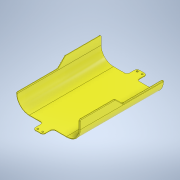
# Autodesk Inventor part: Cover_Inferior
Saved by Autodesk Inventor 2020 (Build 240168000, 168)
## iProperties
Created: 2021-06-25
Part Number: Cover_Inferior
Material: Plástico PC/ABS
Document SubType Name: Modeling
Designer: JCarlos
Density: 0.357273 g/cm^3
Appearance: Amarelo
Author: JCarlos
Autodesk Inventor part; units mm, degrees
ref_plane "YZ Plane" through (0, 0, 0) normal (1, 0, 0) x (0, 1, 0)
ref_plane "XZ Plane" through (0, 0, 0) normal (0, 1, 0) x (-1, 0, 0)
ref_plane "XY Plane" through (0, 0, 0) normal (0, 0, 1) x (1, 0, 0)
sketch "Esboço1" plane through (0, 0, 0) normal (0, 0, 1) x (1, 0, 0)
  line L0 (-62.5, 0) -> (-62.5, -10)
  line L1 (-37.5, -35) -> (37.5, -35)
  line L2 (62.5, -10) -> (62.5, 0)
  arc A0 (37.5, -35) -> (62.5, -10) centre (37.5, -10) ccw
  arc A1 (-62.5, -10) -> (-37.5, -35) centre (-37.5, -10) ccw
  line L3 (37.5, -37) -> (-37.5, -37)
  arc A2 (-64.5, -10) -> (-37.5, -37) centre (-37.5, -10) ccw
  line L4 (-64.5, -10) -> (-64.5, 0)
  line L5 (64.5, 0) -> (64.5, -10)
  arc A3 (37.5, -37) -> (64.5, -10) centre (37.5, -10) ccw
  line L6 (-64.5, 0) -> (-62.5, 0)
  line L7 (62.5, 0) -> (64.5, 0)
  point P0 (0, 0)
  point P1 (0, 0)
  point P2 (0, -35)
  dimension "d0" = 125
  dimension "d2" = 25
  dimension "d21" = 2
  dimension "d22" = 37
  dimension "d23" = 2
  dimension "d24" = 2
  dimension "d25" = 2
  dimension "d26" = 2
  constraints: 16 end point, 8 point on circle, 4 centre point, 4 tangent, 2 horizontal, 2 perpendicular, 1 coincident, 1 collinear, 1 equal radius, 1 horizontal alignment, 1 midpoint, 1 vertical alignment, 1 other
  measures "d0" distance between parallel lines of L0 L2
  measures "d2" radius of A0
  measures "d21" distance between parallel lines of L1 L3
  measures "d22" distance between parallel lines of L3 L6
  measures "d23" distance between parallel lines of L0 L4
  measures "d24" distance between parallel lines of L2 L5
  measures "d25" radial gap between concentric circles of A3 A0
  measures "d26" radial gap between concentric circles of A2 A1
extrude "Extrusão1" add sketch "Esboço1" along normal mid plane 170
sketch "Esboço2" plane through (64.5, -10, 85) normal (1, 0, 0) x (0, 0, -1)
  line L0 (0, 10) -> (0, 0) projected
  line L1 (0, 10) -> (0, 17.5)
  line L2 (0, 17.5) -> (70.7574, 17.5)
  line L3 (72.8787, 16.6213) -> (86.1213, 3.3787)
  line L4 (88.2426, 2.5) -> (170, 2.5)
  line L5 (170, 0) -> (170, 10) projected
  line L6 (0, 10) -> (170, 10)
  line L7 (170, 2.5) -> (170, 10)
  arc A0 (72.8787, 16.6213) -> (70.7574, 17.5) centre (70.7574, 14.5) ccw
  arc A1 (86.1213, 3.3787) -> (88.2426, 2.5) centre (88.2426, 5.5) ccw
  point P0 (85, 10)
  point P1 (72, 17.5)
  point P2 (79.5, 10)
  dimension "d29" = 7.5
  dimension "d30" = 7.5
  dimension "d31" = 135
  dimension "d32" = 72
  dimension "d33" = 3
  constraints: 12 end point, 4 point on circle, 4 tangent, 3 point on line, 2 centre point, 2 vertical, 1 equal radius, 1 horizontal, 1 parallel, 1 perpendicular
  measures "d29" distance between parallel lines of L6 L2
  measures "d30" distance between parallel lines of L6 L4
  measures "d31" angle of L4 L3
  measures "d32" distance of point (72, 17.5) L1.end
  measures "d33" radius of A0
extrude "Extrusão2" add sketch "Esboço2" against normal up to surface (2 mm away) contours L1 L2 A0 L3 L6
extrude "Extrusão3" cut sketch "Esboço2" against normal up to surface (2 mm away) contours L6 L5 L4 A1 L3
sketch "Esboço3" plane through (-64.5, -10, 85) normal (-1, 0, 0) x (0, 0, 1)
  line L0 (-170, 10) -> (-170, 0) projected
  line L1 (-170, 10) -> (-170, 17.5)
  line L2 (-170, 17.5) -> (-99.2426, 17.5)
  line L3 (-97.1213, 16.6213) -> (-83.8787, 3.3787)
  line L4 (-81.7574, 2.5) -> (0, 2.5)
  line L5 (0, 17.5) -> (0, 0) projected
  line L6 (-170, 10) -> (0, 10) projected
  line L7 (0, 10) -> (-170, 10)
  arc A0 (-97.1213, 16.6213) -> (-99.2426, 17.5) centre (-99.2426, 14.5) ccw
  arc A1 (-83.8787, 3.3787) -> (-81.7574, 2.5) centre (-81.7574, 5.5) ccw
  line L8 (0, 2.5) -> (0, 10)
  line L9 (-70.7574, 17.5) -> (0, 17.5) projected
  line L10 (-88.2426, 2.5) -> (-170, 2.5) projected
  point P0 (-85, 10)
  point P1 (-98, 17.5)
  point P2 (-90.5, 10)
  dimension "d41" = 72
  dimension "d42" = 3
  dimension "d56" = 135
  constraints: 12 end point, 4 collinear, 4 point on circle, 4 tangent, 3 point on line, 2 centre point, 1 equal radius, 1 parallel, 1 perpendicular, 1 vertical
  measures "d41" distance of point (-98, 17.5) L1.end
  measures "d42" radius of A0
  measures "d56" angle of L4 L3
extrude "Extrusão4" add sketch "Esboço3" against normal up to surface (2 mm away) contours L1 L2 A0 L3 L6
extrude "Extrusão5" cut sketch "Esboço3" against normal up to surface (2 mm away) contours L6 L5 L4 A1 L3
sketch "Esboço4" plane through (-37.5, -37, 85) normal (0, -1, 0) x (1, 0, 0)
  line L0 (47.5, -170) -> (27.5, -170)
  line L1 (27.5, -170) -> (27.5, -190)
  line L2 (27.5, -190) -> (47.5, -190)
  line L3 (47.5, -190) -> (47.5, -170)
  line L4 (75, -170) -> (0, -170) projected
  point P0 (37.5, -85)
  point P1 (37.5, -190)
  dimension "d47" = 20
  dimension "d48" = 20
  constraints: 8 end point, 2 parallel, 1 collinear, 1 horizontal, 1 midpoint, 1 perpendicular, 1 vertical alignment
  measures "d47" distance of L2.end L0.start
  measures "d48" distance of L1.end L2.end
extrude "Extrusão6" add sketch "Esboço4" against normal up to surface (2 mm away)
sketch "Esboço5" plane through (-37.5, -37, 85) normal (0, -1, 0) x (1, 0, 0)
  circle A0 centre (42.5, -185.5) radius 1.75 projected
  circle A1 centre (32.5, -185.5) radius 1.75 projected
  point P0 (37.5, -85)
extrude "Extrusão7" cut sketch "Esboço5" against normal through all
mirror "Espelhamento1" about plane through (0, 0, 0) normal (0, 0, 1) of "Extrusão6", "Extrusão7"
fillet "Arredondamento1" radius 5 8 edges at (10, -36, 105) (10, -36, 85) (-10, -36, 85) (-10, -36, 105) (10, -36, -85) (10, -36, -105) (-10, -36, -105) (-10, -36, -85)
fillet "Arredondamento2" radius 2.5 4 edges at (63.5, -7.5, -85) (-63.5, 7.5, -85) (63.5, 7.5, 85) (-63.5, -7.5, 85)
fillet "Arredondamento3" radius 1 38 edges at (-11.4645, -37, 86.4645) (-10, -37, 95) (-8.5355, -37, 103.5355) (0, -37, 105) (8.5355, -37, 103.5355) (10, -37, 95) (11.4645, -37, 86.4645) (26.25, -37, 85) (56.5919, -29.0919, 85) (64.5, -2.5, 85) (64.5, 6.7678, 84.2678) (64.5, 7.5, 48.3713) (64.5, 7.2716, 13.0946) (64.5, 0, 5.5) (64.5, -7.2716, -2.0946) (64.5, -7.5, -42.8713) (64.5, -8.2322, -84.2678) (56.5919, -29.0919, -85) (26.25, -37, -85) (11.4645, -37, -86.4645) (10, -37, -95) (8.5355, -37, -103.5355) (0, -37, -105) (-8.5355, -37, -103.5355) (-10, -37, -95) (-11.4645, -37, -86.4645) (-26.25, -37, -85) (-56.5919, -29.0919, -85) (-64.5, -2.5, -85) (-64.5, 6.7678, -84.2678) (-64.5, 7.5, -48.3713) (-64.5, 7.2716, -13.0946) (-64.5, 0, -5.5) (-64.5, -7.2716, 2.0946) (-64.5, -7.5, 42.8713) (-64.5, -8.2322, 84.2678) (-56.5919, -29.0919, 85) (-26.25, -37, 85)
equation "\"d24\" = d23"
equation "\"d30\" = d29"
